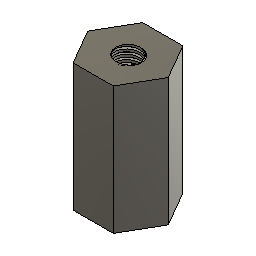
2022-01-30 spacer v1 (Autodesk Fusion 360 design; units mm, degrees)
Autodesk Fusion 360 part; units mm, degrees
note: some values were not read from the file. Set by a fixed rule: the direction of a hole.
sketch "Sketch1" plane through (0, 0, 0) normal (0, 1, 0) x (1, 0, 0)
  line L0 (-1.7321, 3) -> (-3.4641, 0)
  line L1 (-3.4641, 0) -> (-1.7321, -3)
  line L2 (-1.7321, -3) -> (1.7321, -3)
  line L3 (1.7321, -3) -> (3.4641, 0)
  line L4 (3.4641, 0) -> (1.7321, 3)
  line L5 (1.7321, 3) -> (-1.7321, 3)
  dimension "d1" = 6
  measures "d1" distance of L2 L5
extrude "Extrude1" add sketch "Sketch1" along normal blind 11
hole "Hole1" at (0, 0, 0) direction (0, 1, 0) diameter 1.923 depth 12.5 tip angle 118
thread "Thread1" "ISO Metric profile 2.3 M2.3x0.4 6H" major diameter 2.3739 minor diameter 1.923 pitch 0.4 angle 60 modelled right hand crest width 0.1064 on face at (0.0479, 3.6667, -0.9603) crest through (0, 0.1, -0.9615)
sketch "Sketch2" plane through (0, 0, 0) normal (0, 1, 0) x (1, 0, 0)
  circle A0 centre (0, 0) radius 1.05
  dimension "d7" = 2.1
  constraint coincident A0.centre origin
  measures "d7" diameter of A0
extrude "Extrude2" cut sketch "Sketch2" along normal blind 14.3
named bodies: "2022-01-30 spacer"
